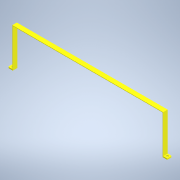
# Autodesk Inventor part: Soporte_Batería2
Saved by Autodesk Inventor 2022.1 (Build 261234000, 234)
## iProperties
Part Number: Soporte_Batería2
Material: Genérico
Document SubType Name: Modelado
Designer: seb_0
Appearance: Amarillo
Author: seb_0
Autodesk Inventor part; units mm, degrees
ref_plane "Plano YZ" through (0, 0, 0) normal (1, 0, 0) x (0, 1, 0)
ref_plane "Plano XZ" through (0, 0, 0) normal (0, 1, 0) x (-1, 0, 0)
ref_plane "Plano XY" through (0, 0, 0) normal (0, 0, 1) x (1, 0, 0)
sketch "Boceto1" plane through (0, 0, 0) normal (0, 1, 0) x (-1, 0, 0)
  line L0 (0, 0) -> (662.2, 0)
  line L1 (662.2, 0) -> (662.2, -20)
  line L2 (662.2, -20) -> (0, -20)
  line L3 (0, -20) -> (0, 0)
  dimension "d0" = 20
  dimension "d1" = 662.2
  constraints: 8 end point, 2 parallel, 1 horizontal, 1 perpendicular
  measures "d0" distance of L2.end L0.start
  measures "d1" distance of L0.start L0.end
extrude "Extrusión1" add sketch "Boceto1" along normal blind 2
sketch "Boceto2" plane through (0, 0, 0) normal (0, -1, 0) x (1, 0, 0)
  line L0 (-662.2, 0) -> (0, 0) projected
  line L1 (0, -20) -> (-662.2, -20) projected
  line L2 (0, 0) -> (-2, 0)
  line L3 (-2, 0) -> (-2, -20)
  line L4 (-2, -20) -> (0, -20)
  line L5 (0, -20) -> (0, 0)
  line L6 (-662.2, 0) -> (-660.2, 0)
  line L7 (-660.2, 0) -> (-660.2, -20)
  line L8 (-660.2, -20) -> (-662.2, -20)
  line L9 (-662.2, -20) -> (-662.2, 0)
  dimension "d4" = 2
  dimension "d5" = 2
  constraints: 16 end point, 4 parallel, 2 horizontal, 2 perpendicular, 2 point on line
  measures "d4" distance between parallel lines of L3 L5
  measures "d5" distance between parallel lines of L9 L7
extrude "Extrusión2" add sketch "Boceto2" along normal blind 165 contours L0 L7 L1 L9 | L0 L5 L1 L3
sketch "Boceto3" plane through (0, -165, 0) normal (0, -1, 0) x (1, 0, 0)
  line L0 (-2, -20) -> (-2, 0) projected
  line L1 (-2, 0) -> (18, 0)
  line L2 (18, 0) -> (18, -20)
  line L3 (18, -20) -> (-2, -20)
  line L4 (-2, -20) -> (-2, 0)
  line L5 (-660.2, 0) -> (-660.2, -20) projected
  line L6 (-660.2, 0) -> (-680.2, 0)
  line L7 (-680.2, 0) -> (-680.2, -20)
  line L8 (-680.2, -20) -> (-660.2, -20)
  line L9 (-660.2, -20) -> (-660.2, 0)
  line L10 (18, 0) -> (-2, -20)
  line L11 (-2, 0) -> (-2, -20) projected
  line L12 (-2, 0) -> (18, -20)
  circle A0 centre (8, -10) radius 5
  line L13 (-660.2, -20) -> (-680.2, 0)
  line L14 (-680.2, -20) -> (-660.2, 0)
  circle A1 centre (-670.2, -10) radius 5
  point P0 (0, 0)
  dimension "d8" = 20
  dimension "d9" = 20
  dimension "d10" = 20
  dimension "d11" = 20
  dimension "d14" = 10
  dimension "d15" = 10
  constraints: 24 end point, 4 parallel, 3 perpendicular, 2 centre point, 2 horizontal, 2 midpoint, 1 point on line
  measures "d8" distance of L1.end L2.end
  measures "d9" distance of L2.end L3.end
  measures "d10" distance of L7.end L8.end
  measures "d11" distance of L6.end L7.end
  measures "d14" diameter of A0
  measures "d15" diameter of A1
extrude "Extrusión3" add sketch "Boceto3" along normal blind 5 contours L10 A0 L12 L3 | L0 L12 A0 L10 | L1 L10 A0 L12 | L12 A0 L10 L2 | L14 A1 L13 L6 | L5 L13 A1 L14 | L8 L14 A1 L13 | L13 A1 L14 L7
fillet "Empalme1" radius 2.5 4 edges at (18, -167.5, 0) (18, -167.5, -20) (-680.2, -167.5, 0) (-680.2, -167.5, -20)
